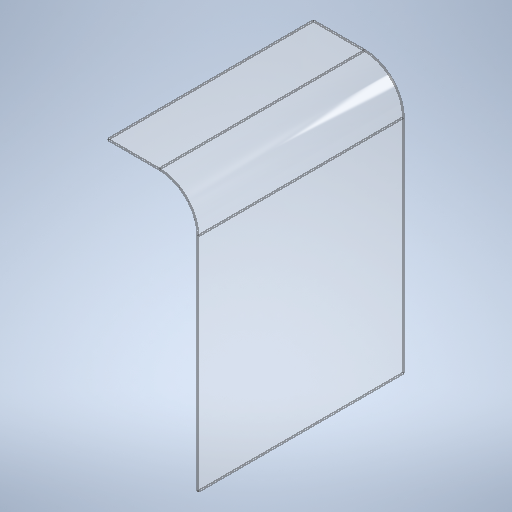
# Autodesk Inventor part: RT_FRM_MC_012_Electrical_housing_door
Saved by Autodesk Inventor 2025.3 (Build 293356000, 356)
## iProperties
Created: 2026-06-06
Part Number: RT_FRM_MC_012_Electrical_housing_door
Material: Polycarbonate, Clear
Document SubType Name: Modeling
Designer: louis
Density: 1.2 g/cm^3
Appearance: Polycarbonate - Clear
Author: louis
Autodesk Inventor part; units mm, degrees
ref_plane "YZ Plane" through (0, 0, 0) normal (1, 0, 0) x (0, 1, 0)
ref_plane "XZ Plane" through (0, 0, 0) normal (0, 1, 0) x (-1, 0, 0)
ref_plane "XY Plane" through (0, 0, 0) normal (0, 0, 1) x (1, 0, 0)
sketch "Sketch1" plane through (0, 0, 0) normal (0, 0, 1) x (1, 0, 0)
  line L0 (-130, 100) -> (0, 100)
  arc A0 (100, 0) -> (0, 100) centre (0, 0) ccw
  line L1 (100, 0) -> (100, -560)
  line L2 (100, -560) -> (96, -560)
  line L3 (96, -560) -> (96, 0)
  arc A1 (96, 0) -> (0, 96) centre (0, 0) ccw
  line L4 (0, 96) -> (-130, 96)
  line L5 (-130, 96) -> (-130, 100)
  dimension "d0" = 4
  dimension "d1" = 660
  dimension "d2" = 230
  dimension "d3" = 100
  constraints: 12 end point, 5 perpendicular, 4 point on circle, 4 tangent, 2 centre point, 1 coincident, 1 concentric, 1 horizontal
  measures "d0" distance of L4.end L0.start
  measures "d1" distance from line of L2.end L0
  measures "d2" horizontal distance of L1.start L0.start
  measures "d3" radius of A0
extrude "Extrusion1" add sketch "Sketch1" along normal mid plane 520
body "Solid1"
